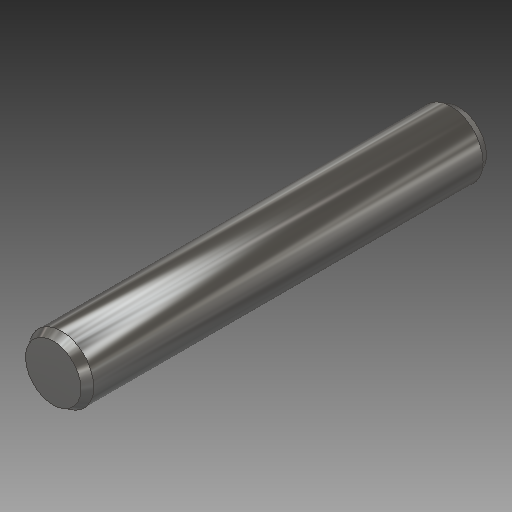
# Autodesk Inventor part: 平行ピンΦ4.25
Saved by Autodesk Inventor 2020 (Build 240168000, 168)
## iProperties
Created: 2018-09-05
Part Number: 平行ピンΦ4.25
Material: 鋼、高強度、低合金
Document SubType Name: Modeling
Designer: 雪村
Density: 7.85 g/cm^3
Appearance: 鋼 - つや出し
Mass: 2.4526 g
Surface Area: 3.33457 cm^2
Volume: 0.312433 cm^3
Author: 雪村
Autodesk Inventor part; units mm, degrees
ref_plane "YZ Plane" through (0, 0, 0) normal (1, 0, 0) x (0, 1, 0)
ref_plane "XZ Plane" through (0, 0, 0) normal (0, 1, 0) x (-1, 0, 0)
ref_plane "XY Plane" through (0, 0, 0) normal (0, 0, 1) x (1, 0, 0)
sketch "スケッチ1" plane through (0, 0, 0) normal (0, 0, 1) x (1, 0, 0)
  circle A0 centre (0, 0) radius 2
  dimension "d0" = 4
  constraints: 1 centre point, 1 coincident
  measures "d0" diameter of A0
extrude "押し出し1" add sketch "スケッチ1" along normal blind 25
chamfer "面取り1" distance 0.5 angle 30 2 edges at (-2, 0, 25) (-2, 0, 0) measured on face at (1.9741, -0.3208, 8.3333)
